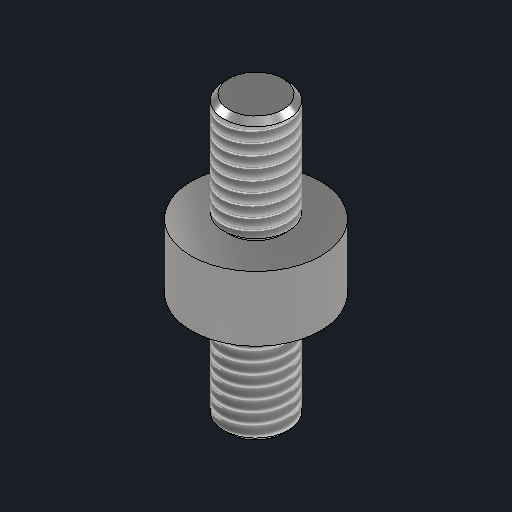
# Autodesk Inventor part: KN-00-02-04
Saved by Autodesk Inventor 2025.2 (Build 292293000, 293)
## iProperties
Created: 2025-04-12
Part Number: KN-00-02-04
Material: X5CrNi18-10
Document SubType Name: Modeling
Designer: Kacper Mik
Density: 8 g/cm^3
Appearance: Semi-Polished
Mass: 15.6786 g
Surface Area: 11.507 cm^2
Volume: 1.95983 cm^3
Author: Kacper Mik
Autodesk Inventor part; units mm, degrees
ref_plane "YZ Plane" through (0, 0, 0) normal (1, 0, 0) x (0, 1, 0)
ref_plane "XZ Plane" through (0, 0, 0) normal (0, 1, 0) x (-1, 0, 0)
ref_plane "XY Plane" through (0, 0, 0) normal (0, 0, 1) x (1, 0, 0)
sketch "Sketch1" plane through (0, 0, 0) normal (0, 1, 0) x (-1, 0, 0)
  circle A0 centre (0, 0) radius 6
  dimension "d0" = 12
  constraints: 1 centre point, 1 coincident
  measures "d0" diameter of A0
extrude "srodek" add sketch "Sketch1" along normal blind 6
sketch "Sketch2" plane through (0, 0, 0) normal (0, -1, 0) x (1, 0, 0)
  circle A0 centre (0, 0) radius 6 projected
  circle A1 centre (0, 0) radius 3
  dimension "d3" = 6
  constraints: 1 centre point, 1 coincident
  measures "d3" diameter of A1
extrude "dolne" add sketch "Sketch2" along normal blind 10 contours A1
thread "Thread1" size "M6x1" class "6g" standard "ANSI Metric M Profile" full length
chamfer "Chamfer1" distance 0.5 angle 45 1 edges at (-3, -10, 0)
sketch "Sketch3" plane through (0, 0, 0) normal (0, 0, 1) x (1, 0, 0)
  line L0 (3, 0) -> (-3, 0) projected
  line L1 (-3, 0) -> (-2.5, 0)
  line L2 (-2.5, 0) -> (-2.5, -0.5)
  line L3 (-2.5, -0.5) -> (-3, -0.5)
  line L4 (-3, -0.5) -> (-3, 0)
  line L5 (0, -0.6) -> (0, 0.1) projected
  point P0 (0, 0)
  point P1 (-2.5, 0)
  dimension "d11" = 0.5
  dimension "d12" = 0.5
  constraints: 8 end point, 2 parallel, 1 horizontal, 1 perpendicular
  measures "d11" distance of L2.end L3.end
  measures "d12" distance of L1.end L2.end
revolve "Revolution1" cut sketch "Sketch3" angle 360 about axis through (0, -10, 0) along (0, 1, 0)
sketch "Sketch6" plane through (0, 6, 0) normal (0, 1, 0) x (1, 0, 0)
  circle A0 centre (0, 0) radius 4 projected
  circle A1 centre (0, 0) radius 3
  dimension "d19" = 6
  constraints: 1 centre point, 1 coincident
  measures "d19" diameter of A1
extrude "mocowanie K1" add sketch "Sketch6" along normal blind 10 contours A1
sketch "Sketch7" plane through (0, 0, 0) normal (1, 0, 0) x (0, 1, 0)
  line L0 (6, -3) -> (6.5, -3)
  line L1 (6.5, -3) -> (6.5, -2.5)
  line L2 (6.5, -2.5) -> (6, -2.5)
  line L3 (6, -2.5) -> (6, -3)
  line L4 (-3.2, 0) -> (19.2, 0) projected
  line L5 (16, -3) -> (16, 3) construction
  line L6 (6, 3) -> (6, -3) construction
  point P0 (0, 0)
  dimension "d27" = 0.5
  dimension "d28" = 0.5
  constraints: 8 end point, 2 parallel, 1 horizontal, 1 perpendicular
  measures "d27" distance of L2.end L1.end
  measures "d28" distance of L1.end L0.end
revolve "Revolution2" cut sketch "Sketch7" angle 360 about axis through (0, -10, 0) along (0, 1, 0)
thread "Thread3" size "M6x1" class "6g" standard "ISO Metric profile" full length
chamfer "Chamfer3" distance 0.5 angle 45 1 edges at (-3, 16, 0)
body "Solid1"
